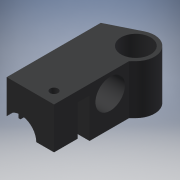
# Autodesk Inventor part: Main_Mirrored
Saved by Autodesk Inventor 2016 SP1 (Build 200210100, 210)
## iProperties
Created: 2015-07-27
Part Number: Main_Mirrored
Material: PLA Plastic
Document SubType Name: Modeling
Designer: Mathias L. Kjeldgaard
Density: 0.996477 g/cm^3
Appearance: Generic
Mass: 18.0345 g
Surface Area: 93.7881 cm^2
Volume: 18.0983 cm^3
d1: 2,000 mm
d2: 15,000 mm
d3: 25,000 mm
d4: 20,000 mm
d5: 8,000 mm
d6: 42,000 mm
d7: 5,000 mm
d8: 18,000 mm
d10: 15,000 mm
d11: 15,000 mm
d12: 40,000 mm
d13: 25,000 mm
d14: 0,00 deg
d15: 15,000 mm
d16: 15,000 mm
d17: 15,000 mm
d19: 18,000 mm
d20: 9,500 mm
d22: 0,00 deg
d30: 2,000 mm
d38: 3,000 mm
d150: 22,000 mm
d151: 20,000 mm
d152: 0,00 deg
d153: -23,000 mm
d154: 10,000 mm
d155: 10,000 mm
d156: 6,000 mm
d158: 180,00 deg
d160: 0,00 deg
d163: 0,00 deg
d165: 0,00 deg
d167: 0,00 deg
d168: 13,000 mm
d169: 0,00 deg
d170: 6,000 mm
d171: 16,000 mm
d172: 0,000 mm
d176: 4,000 mm
d177: 0,00 deg
d179: 0,00 deg
d180: 4,000 mm
d181: 6,000 mm
d182: 6,000 mm
d184: 0,00 deg
d185: 3,000 mm
d186: 0,00 deg
Author: Mathias L. Kjeldgaard
Title: XY-Glider
Autodesk Inventor part; units mm, degrees
ref_plane "YZ Plane" through (0, 0, 0) normal (1, 0, 0) x (0, 1, 0)
ref_plane "XZ Plane" through (0, 0, 0) normal (0, 1, 0) x (-1, 0, 0)
ref_plane "XY Plane" through (0, 0, 0) normal (0, 0, 1) x (1, 0, 0)
sketch "Sketch1" plane through (0, 0, 0) normal (0, 0, 1) x (1, 0, 0)
  circle A0 centre (11.9875, 17.6045) radius 7.5
  arc A1 (18.7629, 10.9455) -> (7.7868, 26.1253) centre (11.9875, 17.6045) ccw
  line L0 (-8.0125, -7.3955) -> (-0.0125, -7.3955) construction
  line L1 (-0.0125, -7.3955) -> (-0.0125, 4.8295) construction
  line L2 (16.9875, 9.139) -> (16.9875, -32.861)
  line L3 (16.9875, -32.861) -> (-23.0125, -32.861)
  line L4 (-23.0125, -32.861) -> (-23.0125, 10.9414)
  line L5 (37.2097, -0.3955) -> (-34.0078, -0.3955) construction
  line L6 (31.0948, -7.8955) -> (-30.4036, -7.8955) construction
  line L7 (29.7312, 7.1045) -> (-30.4036, 7.1045) construction
  line L8 (-23.0125, 10.9414) -> (7.7868, 26.1253)
  line L9 (16.9875, 9.139) -> (18.7629, 10.9455)
  dimension "d1" = 2
  dimension "d2" = 15
  dimension "d3" = 25
  dimension "d4" = 20
  dimension "d5" = 8
  dimension "d6" = 42
  dimension "d7" = 5
  dimension "d8" = 18
  dimension "d10" = 15
  dimension "d11" = 15
  dimension "d12" = 40
  constraints: 20 end point, 3 parallel, 2 centre point, 2 perpendicular, 2 point on circle, 2 tangent, 1 coincident, 1 horizontal
  measures "d1" radial gap between concentric circles of A1 A0
  measures "d2" diameter of A0
  measures "d3" vertical distance of A0.centre L0.start
  measures "d4" horizontal distance of A0.centre L0.start
  measures "d5" distance from line of L0.start L1
  measures "d6" distance of L2.start L2.end
  measures "d7" distance from line of A0.centre L2
  measures "d8" distance from line of A0.centre L5
  measures "d10" diameter of L7 L5
  measures "d11" diameter of L6 L5
  measures "d12" distance between parallel lines of L4 L2
extrude "Extrusion1" add sketch "Sketch1" along normal blind 25
sketch "Sketch2" plane through (-23.0125, -32.861, 0) normal (-1, 0, 0) x (0, 0, 1)
  line L0 (0, 43.8024) -> (0, 0) construction
  line L1 (25, 57.9655) -> (25, 42.9655) construction
  line L2 (0, 42.9655) -> (0, 57.9655) construction
  line L3 (25, 50.4655) -> (0, 50.4655) construction
  line L4 (25, 57.9655) -> (0, 57.9655) construction
  line L5 (25, 42.9655) -> (0, 42.9655) construction
  line L6 (25, 57.9655) -> (25, 42.9655) construction
  line L7 (37.5603, 32.4655) -> (-20.7807, 32.4655) construction
  circle A0 centre (9.5, 32.4655) radius 7.5
  point P0 (0, 32.861)
  dimension "d15" = 15
  dimension "d16" = 15
  dimension "d17" = 15
  dimension "d19" = 18
  dimension "d20" = 9.5
  constraints: 8 end point, 5 point on line, 3 perpendicular, 2 midpoint, 1 centre point
  measures "d15" diameter of L5 L3
  measures "d16" diameter of L4 L3
  measures "d17" diameter of A0
  measures "d19" distance between parallel lines of L3 L7
  measures "d20" distance from line of L0 A0.centre
extrude "Y Glide hul" cut sketch "Sketch2" against normal up to surface (40 mm away)
sketch "Sketch25" plane through (0, 0, 25) normal (0, 0, 1) x (1, 0, 0)
  line L0 (-23.0125, -32.861) -> (16.9875, -32.861) projected
  line L1 (-23.0125, 10.9414) -> (-23.0125, -32.861) projected
  line L2 (16.9875, -32.861) -> (-23.0125, -32.861)
  line L3 (-23.0125, -32.861) -> (-23.0125, -10.861)
  line L4 (-23.0125, -10.861) -> (16.9875, -10.861)
  line L5 (16.9875, -10.861) -> (16.9875, -32.861)
  dimension "d150" = 22
  constraints: 8 end point, 2 parallel, 1 horizontal, 1 perpendicular, 1 point on line
  measures "d150" distance between parallel lines of L2 L4
extrude "Extrusion23" cut sketch "Sketch25" against normal blind 20
ref_plane "Work Plane7" through (-0.0125, -32.861, 0) normal (-1, 0, 0) x (0, 0, 1)
sketch "Sketch29" plane through (-0.0125, -32.861, 0) normal (-1, 0, 0) x (0, 0, 1)
  line L0 (5, 22) -> (25, 22) construction
  line L1 (25, 43.8024) -> (25, 22) construction
  line L2 (0, 43.8024) -> (25, 43.8024) construction
  line L3 (0, 43.8024) -> (0, 0) construction
  line L4 (0, 0) -> (5, 0) construction
  line L5 (5, 0) -> (5, 22) construction
  circle A0 centre (9.5, 32.4655) radius 7.5 construction
  line L6 (5, 22) -> (5, 0) projected
  line L7 (5, 0) -> (5, 10)
  line L8 (5, 10) -> (15, 10)
  line L9 (15, 10) -> (15, 16)
  line L10 (15, 16) -> (5, 16)
  line L11 (21, 3) -> (21, 19.5032) construction
  point P0 (0, 32.861)
  dimension "d154" = 10
  dimension "d155" = 10
  dimension "d156" = 6
  dimension "d170" = 6
  constraints: 10 end point, 3 perpendicular, 2 point on line, 1 vertical
  measures "d154" distance of L4.end L7.end
  measures "d155" distance of L7.end L8.end
  measures "d156" distance between parallel lines of L10 L8
  measures "d170" distance between parallel lines of L11 L9
revolve "Revolution2" add sketch "Sketch29" angle 180 mid plane about axis through (-0.0125, -29.861, 21) along (0, 1, 0)
sketch "Sketch30" plane through (5.9875, -22.861, 21) normal (0, -1, 0) x (1, 0, 0)
  line L0 (10, 0) -> (0, 0) projected
  arc A0 (-12, 0) -> (0, 0) centre (-6, 0) ccw projected
  line L1 (-22, 0) -> (-12, 0) projected
  arc A1 (-22, 0) -> (-6, -16) centre (-6, 0) ccw projected
  arc A2 (-6, -16) -> (10, 0) centre (-6, 0) ccw projected
  arc A3 (-12, 0) -> (0, 0) centre (-6, 0) ccw
  line L2 (10, 0) -> (0, 0) projected
  line L3 (10, 0) -> (0, 0)
  line L4 (-12, 0) -> (-22, 0)
  line L5 (11, -16) -> (-29, -16) projected
  line L6 (-29, -21) -> (-29, -16) projected
  line L7 (-29, -21) -> (11, -21) projected
  line L8 (11, -21) -> (11, -16) projected
  line L9 (-22, 0) -> (-22, -16)
  line L10 (-22, -16) -> (-6, -16)
  line L11 (10, 0) -> (10, -16)
  line L12 (10, -16) -> (-6, -16)
  point P0 (-5.9875, -21)
  constraints: 16 end point, 3 collinear, 2 perpendicular, 2 point on circle, 2 point on line, 1 centre point, 1 concentric, 1 horizontal, 1 tangent
extrude "Extrusion24" add sketch "Sketch30" against normal up to surface (6 mm away) contours A2 A1 L1 A0 L0 | L11 L5 A2 | L5 L9 A1
sketch "Sketch32" plane through (-0.0125, -22.861, 21) normal (0, -1, 0) x (1, 0, 0)
  line L0 (16, 0) -> (6, 0) projected
  arc A0 (-6, 0) -> (6, 0) centre (0, 0) ccw projected
  line L1 (-16, 0) -> (-6, 0) projected
  line L2 (-16, 0) -> (-16, -16) projected
  line L3 (16, -16) -> (-16, -16) projected
  line L4 (16, -16) -> (16, 0) projected
  line L5 (16, -16) -> (16, 0) projected
  line L6 (16, 0) -> (16, -16)
  line L7 (16, -16) -> (-3, -16)
  line L8 (-23, -16) -> (17, -16) projected
  line L9 (-16, 0) -> (-16, -16) projected
  line L10 (-3, -16) -> (-16, -16)
  line L11 (-16, -16) -> (-16, 0)
  arc A1 (-8, 0) -> (8, 0) centre (0, 0) ccw
  line L12 (6, 0) -> (16, 0) projected
  line L13 (16, -16) -> (16, 0) projected
  line L14 (-16, -16) -> (16, -16) projected
  line L15 (-16, 0) -> (-16, -16) projected
  line L16 (-6, 0) -> (-16, 0) projected
  arc A2 (-6, 0) -> (6, 0) centre (0, 0) ccw projected
  point P0 (0.0125, -21)
  dimension "d171" = 16
  constraints: 8 end point, 2 point on circle, 2 point on line, 1 centre point, 1 coincident, 1 horizontal, 1 midpoint, 1 perpendicular, 1 vertical
  measures "d171" diameter of A1
extrude "Extrusion25" add sketch "Sketch32" along normal up to surface (10 mm away) contours L4 L3 L2 L1 A1 L0
sketch "Sketch35" plane through (15.9875, -32.861, 5) normal (1, 0, 0) x (0, 0, -1)
  line L0 (0, 16) -> (-16, 16) projected
  line L1 (-16, 16) -> (-16, 0) projected
  line L2 (-16, 0) -> (0, 0) projected
  line L3 (0, 16) -> (0, 0) projected
  line L4 (-13, 7) -> (-13, 0) projected
  line L5 (-13, 0) -> (0, 0)
  line L6 (0, 0) -> (0, 16)
  line L7 (0, 16) -> (-13, 16)
  line L8 (-13, 16) -> (-13, 0)
  point P0 (5, 32.861)
  constraints: 8 end point, 2 parallel, 1 horizontal, 1 perpendicular
extrude "Extrusion26" add sketch "Sketch35" along normal up to surface (1 mm away) contours L3 L2 L4 L8 L0
sketch "Sketch36" plane through (-16.0125, -32.861, 5) normal (-1, 0, 0) x (0, 0, 1)
  line L0 (16, 16) -> (0, 16) projected
  line L1 (0, 0) -> (0, 16) projected
  line L2 (0, 0) -> (16, 0) projected
  line L3 (16, 16) -> (16, 0) projected
  line L4 (16, 10) -> (16, 16) projected
  line L5 (16, 16) -> (0, 16)
  line L6 (0, 16) -> (0, 0)
  line L7 (0, 0) -> (16, 0)
  line L8 (16, 0) -> (16, 16)
  point P0 (-5, 32.861)
  constraints: 8 end point, 2 parallel, 1 horizontal, 1 perpendicular
extrude "Extrusion27" add sketch "Sketch36" along normal up to surface (7 mm away)
sketch "Sketch38" plane through (-23.0125, -32.861, 0) normal (-1, 0, 0) x (0, 0, 1)
  line L0 (5, 22) -> (25, 22) projected
  line L1 (25, 43.8024) -> (25, 22) projected
  line L2 (0, 43.8024) -> (25, 43.8024) projected
  line L3 (0, 43.8024) -> (0, 0) projected
  line L4 (0, 0) -> (21, 0) projected
  line L5 (21, 16) -> (21, 0) projected
  line L6 (5, 16) -> (21, 16) projected
  line L7 (5, 16) -> (5, 22) projected
  circle A0 centre (9.5, 32.4655) radius 7.5 projected
  line L8 (0, 43.8024) -> (25, 43.8024) projected
  line L9 (0, 43.8024) -> (0, 64.0171)
  line L10 (0, 64.0171) -> (25, 64.0171)
  line L11 (25, 64.0171) -> (25, 43.8024)
  line L12 (5, 43.8024) -> (0, 43.8024)
  line L13 (25, 43.8024) -> (0, 43.8024)
  point P0 (0, 32.861)
  constraints: 10 end point, 2 parallel, 1 collinear, 1 horizontal, 1 perpendicular, 1 point on line
extrude "Extrusion28" cut sketch "Sketch38" against normal blind 13
ref_plane "Work Plane8" through (-0.0125, -16.861, 21) normal (0, 1, 0) x (1, 0, 0)
sketch "Sketch40" plane through (7.9875, -32.861, 21) normal (0, -1, 0) x (1, 0, 0)
  line L0 (-18, 0) -> (-18, -21) projected
  line L1 (-18, -21) -> (9, -21) projected
  line L2 (9, -21) -> (9, -3) projected
  line L3 (8, -3) -> (9, -3) projected
  line L4 (8, 0) -> (8, -3) projected
  line L5 (0, 0) -> (8, 0) projected
  arc A0 (-16, 0) -> (0, 0) centre (-8, 0) ccw projected
  line L6 (-18, 0) -> (-16, 0) projected
  point P0 (-7.9875, -21)
extrude "Extrusion30" cut sketch "Sketch40" against normal blind 4
sketch "Sketch41" plane through (15.9875, -16.861, 18) normal (0, 0, 1) x (1, 0, 0)
  line L0 (0, -12) -> (1, -12) projected
  line L1 (1, -12) -> (1, 0) projected
  line L2 (0, 0) -> (1, 0) projected
  line L3 (0, -12) -> (0, 0) projected
  point P0 (-15.9875, 16.861)
extrude "Extrusion31" add sketch "Sketch41" along normal up to surface (3 mm away)
sketch "Sketch42" plane through (5.9875, -16.861, 21) normal (0, 0, 1) x (1, 0, 0)
  circle A0 centre (5, -6) radius 2
  line L0 (0, 0) -> (11, 0) projected
  line L1 (11, 0) -> (11, -12) projected
  point P0 (-5.9875, 16.861)
  dimension "d180" = 4
  dimension "d181" = 6
  dimension "d182" = 6
  constraints: 1 centre point
  measures "d180" diameter of A0
  measures "d181" distance from line of L0 A0.centre
  measures "d182" distance from line of L1 A0.centre
extrude "Holder montering" cut sketch "Sketch42" against normal up to surface (21 mm away)
sketch "Sketch43" plane through (-10.0125, -32.861, 0) normal (-1, 0, 0) x (0, 0, 1)
  circle A0 centre (9.5, 32.4655) radius 7.5 projected
  line L0 (0, 4) -> (21, 4) projected
  line L1 (21, 16) -> (21, 4) projected
  line L2 (5, 16) -> (21, 16) projected
  line L3 (5, 22) -> (5, 16) projected
  line L4 (25, 22) -> (5, 22) projected
  line L5 (25, 50.2113) -> (25, 22) projected
  line L6 (0, 50.2113) -> (25, 50.2113) construction
  line L7 (0, 4) -> (0, 50.2113) projected
  line L8 (25, 50.2113) -> (25, 62.2894)
  line L9 (25, 62.2894) -> (0, 62.2894)
  line L10 (0, 50.2113) -> (25, 50.2113) construction
  line L11 (0, 62.2894) -> (0, 50.2113)
  point P0 (0, 32.861)
  constraints: 6 end point, 2 perpendicular, 1 vertical
extrude "Extrusion33" cut sketch "Sketch43" against normal blind 3
mirror "Mirror1" about plane through (-1.5514, -6.5733, 0) normal (0, 0, -1) remove original yes
equation "\"d11\" = d10"
equation "\"d16\" = d15"
body "Solid1"
